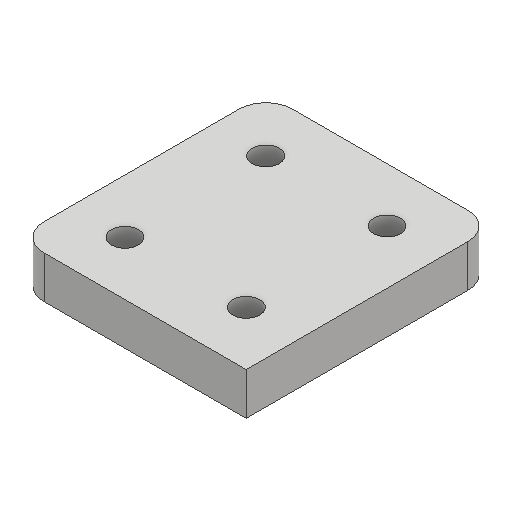
# Autodesk Inventor part: 3DP_ABS_Induction_Sensor_Mount_Spacer
Saved by Autodesk Inventor 2026.1 (Build 301233000, 233)
## iProperties
Created: 2017-05-27
Part Number: 3DP_ABS_Induction_Sensor_Mount_Spacer
Material: Ogólny
Document SubType Name: Modeling
Designer: Andrzej
Density: 1 g/cm^3
Appearance: Domyślna
Mass: 3.15673 g
Surface Area: 20.0216 cm^2
Volume: 3.15673 cm^3
Author: Andrzej
Autodesk Inventor part; units mm, degrees
ref_plane "YZ Plane" through (0, 0, 0) normal (1, 0, 0) x (0, 1, 0)
ref_plane "XZ Plane" through (0, 0, 0) normal (0, 1, 0) x (-1, 0, 0)
ref_plane "XY Plane" through (0, 0, 0) normal (0, 0, 1) x (1, 0, 0)
sketch "Szkic1" plane through (0, 0, 0) normal (0, 0, 1) x (1, 0, 0)
  arc A0 (18.7419, 4.0884) -> (15.7419, 7.0884) centre (15.7419, 4.0884) ccw
  line L0 (15.7419, 7.0884) -> (-3.7581, 7.0884)
  arc A1 (-3.7581, 7.0884) -> (-6.7581, 4.0884) centre (-3.7581, 4.0884) ccw
  line L1 (-6.7581, 4.0884) -> (-6.7581, -17.5866)
  arc A2 (-6.7581, -17.5866) -> (-3.7581, -20.5866) centre (-3.7581, -17.5866) ccw
  line L2 (-3.7581, -20.5866) -> (18.7419, -20.5866)
  line L3 (18.7419, -20.5866) -> (18.7419, 4.0884)
  circle A3 centre (12.7419, -14.5866) radius 1.5
  circle A4 centre (12.7419, 1.0884) radius 1.5
  circle A5 centre (-0.7581, 1.0884) radius 1.5
  circle A6 centre (-0.7581, -14.5866) radius 1.5
  point P0 (0, 0)
  point P1 (0, 0)
  constraints: 8 end point, 7 centre point, 6 point on circle
extrude "Wyciągnięcie proste1" add sketch "Szkic1" along normal blind 4.7
